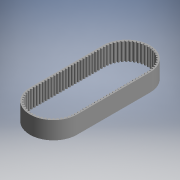
# Autodesk Inventor part: SLZ_63_Riemen#
Saved by Autodesk Inventor 2017.3 (Build 213256000, 256)
## iProperties
Part Number: SLZ_63_Riemen#
Material: Generic
Catalog Web Link: www.cadenas.de
Description: Riemen_SLZ63-Control-Tec
Vendor: ROSEKRIEGER
Document SubType Name: Modeling
Designer: partserver
Manufacturer: ROSEKRIEGER
Mass: 50.6703 g
Surface Area: 430.175 cm^2
Volume: 50.6703 cm^3
Density: 1 g/cm^3
Appearance: PSOLRGB-191-191-191
Category: PARTsolutions
Company: ROSEKRIEGER
Title: SLZ_63_Riemen#
Author: Cadenas PARTsolutions
Comments: Control-Tec
PSOL_IDENT_0: {$CADENAS_DATA\23d-libs\rose_krieger\linearkomponenten\pool_lineartechnik\_hubsaeule_zyliinder\elekt
PSOL_IDENT_1: rozylinder\elekzyl_slz63\parts\slz63_plfl_antrieb_riemen.prj},174 {VTYP=3D},{NB=SLZ_63_Riemen#},{LIN
PSOL_IDENT_2: A=SLZ_63_Riemen#},{NN=Riemen_SLZ63},{DATE=02.12.2020 11:16:24},{GEOMDATE=22.06.2016 13:11:00},{VERSI
PSOL_IDENT_3: ON=},{LINEID=10},{WBVAR=},{WBNUMERIC=}  {NB=SLZ_63_Riemen#},{LINA=SLZ_63_Riemen#},{KT=DUMMY},{IDNR=}
PSOL_IDENT_4: ,{CODE=TQ3},{ARTIKEL=Elektrozylinder },{TYPE=SLZ 63 KG P PL},{BEST=SLZ_63_Riemen},{VARIANTE=PL},{SPI
PSOL_IDENT_5: NDEL=KG 25x10},{SPINDELCODE=3.000},{SCHUTZARTVIS=IP54},{SCHUTZART=1},{HUB1=0,[0:100]},{HINWEINBAUX=H
PSOL_IDENT_6: ub + 288,5 mm},{DUMMYDURCH=10.000},{DUMMYLAENG=20.000},{HILFEHUB=105},{LAENDOPPROFIL=184.500},{RF=1.
PSOL_IDENT_7: 000},{GRUNDKOE=288.500},{A=100},{B=80},{C=100},{D=125},{E=238},{F=40},{G=M16x1.5},{H=104},{K=125},{L=
PSOL_IDENT_8: 105},{M=48},{N=56.5},{O=86},{P=18.5},{PPATH=sbl_lz70p_plfl.prj}
NB: SLZ_63_Riemen#
NN: Riemen_SLZ63
NT: Control-Tec
NBSYN: $BEST.#
LINA: SLZ_63_Riemen#
CATALOG: RK Rose+Krieger
ARTIKEL: Elektrozylinder
TYPE: SLZ 63 KG P PL
BEST: SLZ_63_Riemen
VARIANTE: PL
SPINDEL: KG 25x10
SPINDELCODE: 3
SCHUTZARTVIS: IP54
SCHUTZART: 1
HUB1: 0,[0:100]
HINWEINBAUX: Hub + 288,5 mm
DUMMYDURCH: 10
DUMMYLAENG: 20
HILFEHUB: 105
LAENDOPPROFIL: 184.5
RF: 1
GRUNDKOE: 288.5
A: 100
B: 80
C: 100
D: 125
E: 238
F: 40
G: M16x1.5
H: 104
K: 125
L: 105
M: 48
N: 56.5
O: 86
P: 18.5
SUPPLIER: ROSEKRIEGER
ARTICLENO: SLZ_63_Riemen#
BOMINFO: SLZ_63_Riemen#
CREATOR: CADENAS GmbH
Autodesk Inventor part; units mm, degrees
sketch "Sketch_2" plane through (0, 0, 0) normal (0, 0, 1) x (1, 0, 0)
  arc A0 (-40.2, -125) -> (40.2, -125) centre (0, -125) ccw
  line L0 (40.2, -125) -> (40.2, 0)
  arc A1 (40.2, 0) -> (-40.2, 0) centre (0, 0) ccw
  line L1 (-40.2, 0) -> (-40.2, -125)
  arc A2 (-38.1613, -126.7182) -> (-38.195, -123.2926) centre (-37.625, -125) ccw
  arc A3 (-38.1613, -126.7182) -> (-38.0591, -128.2775) centre (0, -125) ccw
  arc A4 (-37.6106, -131.6846) -> (-38.0591, -128.2775) centre (-37.3031, -129.911) ccw
  arc A5 (-37.6106, -131.6846) -> (-37.3057, -133.2172) centre (0, -125) ccw
  arc A6 (-36.4163, -136.5366) -> (-37.3057, -133.2172) centre (-36.343, -134.7381) ccw
  arc A7 (-36.4163, -136.5366) -> (-35.914, -138.0163) centre (0, -125) ccw
  arc A8 (-34.5989, -141.1912) -> (-35.914, -138.0163) centre (-34.761, -139.3985) ccw
  arc A9 (-34.5989, -141.1912) -> (-33.9078, -142.5926) centre (0, -125) ccw
  arc A10 (-32.1896, -145.5687) -> (-33.9078, -142.5926) centre (-32.5842, -143.8125) ccw
  arc A11 (-32.1896, -145.5687) -> (-31.3214, -146.868) centre (0, -125) ccw
  arc A12 (-29.2294, -149.5943) -> (-31.3214, -146.868) centre (-29.8499, -147.9046) ccw
  arc A13 (-29.2294, -149.5943) -> (-28.1991, -150.7692) centre (0, -125) ccw
  arc A14 (-25.7692, -153.1991) -> (-28.1991, -150.7692) centre (-26.6049, -151.6049) ccw
  arc A15 (-25.7692, -153.1991) -> (-24.5943, -154.2294) centre (0, -125) ccw
  arc A16 (-21.868, -156.3214) -> (-24.5943, -154.2294) centre (-22.9046, -154.8499) ccw
  arc A17 (-21.868, -156.3214) -> (-20.5687, -157.1896) centre (0, -125) ccw
  arc A18 (-17.5926, -158.9078) -> (-20.5687, -157.1896) centre (-18.8125, -157.5842) ccw
  arc A19 (-17.5926, -158.9078) -> (-16.1912, -159.5989) centre (0, -125) ccw
  arc A20 (-13.0163, -160.914) -> (-16.1912, -159.5989) centre (-14.3985, -159.761) ccw
  arc A21 (-13.0163, -160.914) -> (-11.5366, -161.4163) centre (0, -125) ccw
  arc A22 (-8.2172, -162.3057) -> (-11.5366, -161.4163) centre (-9.7381, -161.343) ccw
  arc A23 (-8.2172, -162.3057) -> (-6.6846, -162.6106) centre (0, -125) ccw
  arc A24 (-3.2775, -163.0591) -> (-6.6846, -162.6106) centre (-4.911, -162.3031) ccw
  arc A25 (-3.2775, -163.0591) -> (-1.7182, -163.1613) centre (0, -125) ccw
  arc A26 (1.7182, -163.1613) -> (-1.7182, -163.1613) centre (0, -162.625) ccw
  arc A27 (1.7182, -163.1613) -> (3.2775, -163.0591) centre (0, -125) ccw
  arc A28 (6.6846, -162.6106) -> (3.2775, -163.0591) centre (4.911, -162.3031) ccw
  arc A29 (6.6846, -162.6106) -> (8.2172, -162.3057) centre (0, -125) ccw
  arc A30 (11.5366, -161.4163) -> (8.2172, -162.3057) centre (9.7381, -161.343) ccw
  arc A31 (11.5366, -161.4163) -> (13.0163, -160.914) centre (0, -125) ccw
  arc A32 (16.1912, -159.5989) -> (13.0163, -160.914) centre (14.3985, -159.761) ccw
  arc A33 (16.1912, -159.5989) -> (17.5926, -158.9078) centre (0, -125) ccw
  arc A34 (20.5687, -157.1896) -> (17.5926, -158.9078) centre (18.8125, -157.5842) ccw
  arc A35 (20.5687, -157.1896) -> (21.868, -156.3214) centre (0, -125) ccw
  arc A36 (24.5943, -154.2294) -> (21.868, -156.3214) centre (22.9046, -154.8499) ccw
  arc A37 (24.5943, -154.2294) -> (25.7692, -153.1991) centre (0, -125) ccw
  arc A38 (28.1991, -150.7692) -> (25.7692, -153.1991) centre (26.6049, -151.6049) ccw
  arc A39 (28.1991, -150.7692) -> (29.2294, -149.5943) centre (0, -125) ccw
  arc A40 (31.3214, -146.868) -> (29.2294, -149.5943) centre (29.8499, -147.9046) ccw
  arc A41 (31.3214, -146.868) -> (32.1896, -145.5687) centre (0, -125) ccw
  arc A42 (33.9078, -142.5926) -> (32.1896, -145.5687) centre (32.5842, -143.8125) ccw
  arc A43 (33.9078, -142.5926) -> (34.5989, -141.1912) centre (0, -125) ccw
  arc A44 (35.914, -138.0163) -> (34.5989, -141.1912) centre (34.761, -139.3985) ccw
  arc A45 (35.914, -138.0163) -> (36.4163, -136.5366) centre (0, -125) ccw
  arc A46 (37.3057, -133.2172) -> (36.4163, -136.5366) centre (36.343, -134.7381) ccw
  arc A47 (37.3057, -133.2172) -> (37.6106, -131.6846) centre (0, -125) ccw
  arc A48 (38.0591, -128.2775) -> (37.6106, -131.6846) centre (37.3031, -129.911) ccw
  arc A49 (38.0591, -128.2775) -> (38.1613, -126.7182) centre (0, -125) ccw
  arc A50 (38.195, -123.2926) -> (38.1613, -126.7182) centre (37.625, -125) ccw
  line L2 (38.195, -123.2926) -> (38.195, -121.7074)
  arc A51 (38.195, -118.2926) -> (38.195, -121.7074) centre (37.625, -120) ccw
  line L3 (38.195, -118.2926) -> (38.195, -116.7074)
  arc A52 (38.195, -113.2926) -> (38.195, -116.7074) centre (37.625, -115) ccw
  line L4 (38.195, -113.2926) -> (38.195, -111.7074)
  arc A53 (38.195, -108.2926) -> (38.195, -111.7074) centre (37.625, -110) ccw
  line L5 (38.195, -108.2926) -> (38.195, -106.7074)
  arc A54 (38.195, -103.2926) -> (38.195, -106.7074) centre (37.625, -105) ccw
  line L6 (38.195, -103.2926) -> (38.195, -101.7074)
  arc A55 (38.195, -98.2926) -> (38.195, -101.7074) centre (37.625, -100) ccw
  line L7 (38.195, -98.2926) -> (38.195, -96.7074)
  arc A56 (38.195, -93.2926) -> (38.195, -96.7074) centre (37.625, -95) ccw
  line L8 (38.195, -93.2926) -> (38.195, -91.7074)
  arc A57 (38.195, -88.2926) -> (38.195, -91.7074) centre (37.625, -90) ccw
  line L9 (38.195, -88.2926) -> (38.195, -86.7074)
  arc A58 (38.195, -83.2926) -> (38.195, -86.7074) centre (37.625, -85) ccw
  line L10 (38.195, -83.2926) -> (38.195, -81.7074)
  arc A59 (38.195, -78.2926) -> (38.195, -81.7074) centre (37.625, -80) ccw
  line L11 (38.195, -78.2926) -> (38.195, -76.7074)
  arc A60 (38.195, -73.2926) -> (38.195, -76.7074) centre (37.625, -75) ccw
  line L12 (38.195, -73.2926) -> (38.195, -71.7074)
  arc A61 (38.195, -68.2926) -> (38.195, -71.7074) centre (37.625, -70) ccw
  line L13 (38.195, -68.2926) -> (38.195, -66.7074)
  arc A62 (38.195, -63.2926) -> (38.195, -66.7074) centre (37.625, -65) ccw
  line L14 (38.195, -63.2926) -> (38.195, -61.7074)
  arc A63 (38.195, -58.2926) -> (38.195, -61.7074) centre (37.625, -60) ccw
  line L15 (38.195, -58.2926) -> (38.195, -56.7074)
  arc A64 (38.195, -53.2926) -> (38.195, -56.7074) centre (37.625, -55) ccw
  line L16 (38.195, -53.2926) -> (38.195, -51.7074)
  arc A65 (38.195, -48.2926) -> (38.195, -51.7074) centre (37.625, -50) ccw
  line L17 (38.195, -48.2926) -> (38.195, -46.7074)
  arc A66 (38.195, -43.2926) -> (38.195, -46.7074) centre (37.625, -45) ccw
  line L18 (38.195, -43.2926) -> (38.195, -41.7074)
  arc A67 (38.195, -38.2926) -> (38.195, -41.7074) centre (37.625, -40) ccw
  line L19 (38.195, -38.2926) -> (38.195, -36.7074)
  arc A68 (38.195, -33.2926) -> (38.195, -36.7074) centre (37.625, -35) ccw
  line L20 (38.195, -33.2926) -> (38.195, -31.7074)
  arc A69 (38.195, -28.2926) -> (38.195, -31.7074) centre (37.625, -30) ccw
  line L21 (38.195, -28.2926) -> (38.195, -26.7074)
  arc A70 (38.195, -23.2926) -> (38.195, -26.7074) centre (37.625, -25) ccw
  line L22 (38.195, -23.2926) -> (38.195, -21.7074)
  arc A71 (38.195, -18.2926) -> (38.195, -21.7074) centre (37.625, -20) ccw
  line L23 (38.195, -18.2926) -> (38.195, -16.7074)
  arc A72 (38.195, -13.2926) -> (38.195, -16.7074) centre (37.625, -15) ccw
  line L24 (38.195, -13.2926) -> (38.195, -11.7074)
  arc A73 (38.195, -8.2926) -> (38.195, -11.7074) centre (37.625, -10) ccw
  line L25 (38.195, -8.2926) -> (38.195, -6.7074)
  arc A74 (38.195, -3.2926) -> (38.195, -6.7074) centre (37.625, -5) ccw
  line L26 (38.195, -3.2926) -> (38.195, -1.7074)
  arc A75 (38.1613, 1.7182) -> (38.195, -1.7074) centre (37.625, 0) ccw
  arc A76 (38.1613, 1.7182) -> (38.0591, 3.2775) centre (0, 0) ccw
  arc A77 (37.6106, 6.6846) -> (38.0591, 3.2775) centre (37.3031, 4.911) ccw
  arc A78 (37.6106, 6.6846) -> (37.3057, 8.2172) centre (0, 0) ccw
  arc A79 (36.4163, 11.5366) -> (37.3057, 8.2172) centre (36.343, 9.7381) ccw
  arc A80 (36.4163, 11.5366) -> (35.914, 13.0163) centre (0, 0) ccw
  arc A81 (34.5989, 16.1912) -> (35.914, 13.0163) centre (34.761, 14.3985) ccw
  arc A82 (34.5989, 16.1912) -> (33.9078, 17.5926) centre (0, 0) ccw
  arc A83 (32.1896, 20.5687) -> (33.9078, 17.5926) centre (32.5842, 18.8125) ccw
  arc A84 (32.1896, 20.5687) -> (31.3214, 21.868) centre (0, 0) ccw
  arc A85 (29.2294, 24.5943) -> (31.3214, 21.868) centre (29.8499, 22.9046) ccw
  arc A86 (29.2294, 24.5943) -> (28.1991, 25.7692) centre (0, 0) ccw
  arc A87 (25.7692, 28.1991) -> (28.1991, 25.7692) centre (26.6049, 26.6049) ccw
  arc A88 (25.7692, 28.1991) -> (24.5943, 29.2294) centre (0, 0) ccw
  arc A89 (21.868, 31.3214) -> (24.5943, 29.2294) centre (22.9046, 29.8499) ccw
  arc A90 (21.868, 31.3214) -> (20.5687, 32.1896) centre (0, 0) ccw
  arc A91 (17.5926, 33.9078) -> (20.5687, 32.1896) centre (18.8125, 32.5842) ccw
  arc A92 (17.5926, 33.9078) -> (16.1912, 34.5989) centre (0, 0) ccw
  arc A93 (13.0163, 35.914) -> (16.1912, 34.5989) centre (14.3985, 34.761) ccw
  arc A94 (13.0163, 35.914) -> (11.5366, 36.4163) centre (0, 0) ccw
  arc A95 (8.2172, 37.3057) -> (11.5366, 36.4163) centre (9.7381, 36.343) ccw
  arc A96 (8.2172, 37.3057) -> (6.6846, 37.6106) centre (0, 0) ccw
  arc A97 (3.2775, 38.0591) -> (6.6846, 37.6106) centre (4.911, 37.3031) ccw
  arc A98 (3.2775, 38.0591) -> (1.7182, 38.1613) centre (0, 0) ccw
  arc A99 (-1.7182, 38.1613) -> (1.7182, 38.1613) centre (0, 37.625) ccw
  arc A100 (-1.7182, 38.1613) -> (-3.2775, 38.0591) centre (0, 0) ccw
  arc A101 (-6.6846, 37.6106) -> (-3.2775, 38.0591) centre (-4.911, 37.3031) ccw
  arc A102 (-6.6846, 37.6106) -> (-8.2172, 37.3057) centre (0, 0) ccw
  arc A103 (-11.5366, 36.4163) -> (-8.2172, 37.3057) centre (-9.7381, 36.343) ccw
  arc A104 (-11.5366, 36.4163) -> (-13.0163, 35.914) centre (0, 0) ccw
  arc A105 (-16.1912, 34.5989) -> (-13.0163, 35.914) centre (-14.3985, 34.761) ccw
  arc A106 (-16.1912, 34.5989) -> (-17.5926, 33.9078) centre (0, 0) ccw
  arc A107 (-20.5687, 32.1896) -> (-17.5926, 33.9078) centre (-18.8125, 32.5842) ccw
  arc A108 (-20.5687, 32.1896) -> (-21.868, 31.3214) centre (0, 0) ccw
  arc A109 (-24.5943, 29.2294) -> (-21.868, 31.3214) centre (-22.9046, 29.8499) ccw
  arc A110 (-24.5943, 29.2294) -> (-25.7692, 28.1991) centre (0, 0) ccw
  arc A111 (-28.1991, 25.7692) -> (-25.7692, 28.1991) centre (-26.6049, 26.6049) ccw
  arc A112 (-28.1991, 25.7692) -> (-29.2294, 24.5943) centre (0, 0) ccw
  arc A113 (-31.3214, 21.868) -> (-29.2294, 24.5943) centre (-29.8499, 22.9046) ccw
  arc A114 (-31.3214, 21.868) -> (-32.1896, 20.5687) centre (0, 0) ccw
  arc A115 (-33.9078, 17.5926) -> (-32.1896, 20.5687) centre (-32.5842, 18.8125) ccw
  arc A116 (-33.9078, 17.5926) -> (-34.5989, 16.1912) centre (0, 0) ccw
  arc A117 (-35.914, 13.0163) -> (-34.5989, 16.1912) centre (-34.761, 14.3985) ccw
  arc A118 (-35.914, 13.0163) -> (-36.4163, 11.5366) centre (0, 0) ccw
  arc A119 (-37.3057, 8.2172) -> (-36.4163, 11.5366) centre (-36.343, 9.7381) ccw
  arc A120 (-37.3057, 8.2172) -> (-37.6106, 6.6846) centre (0, 0) ccw
  arc A121 (-38.0591, 3.2775) -> (-37.6106, 6.6846) centre (-37.3031, 4.911) ccw
  arc A122 (-38.0591, 3.2775) -> (-38.1613, 1.7182) centre (0, 0) ccw
  arc A123 (-38.195, -1.7074) -> (-38.1613, 1.7182) centre (-37.625, 0) ccw
  line L27 (-38.195, -1.7074) -> (-38.195, -3.2926)
  arc A124 (-38.195, -6.7074) -> (-38.195, -3.2926) centre (-37.625, -5) ccw
  line L28 (-38.195, -6.7074) -> (-38.195, -8.2926)
  arc A125 (-38.195, -11.7074) -> (-38.195, -8.2926) centre (-37.625, -10) ccw
  line L29 (-38.195, -11.7074) -> (-38.195, -13.2926)
  arc A126 (-38.195, -16.7074) -> (-38.195, -13.2926) centre (-37.625, -15) ccw
  line L30 (-38.195, -16.7074) -> (-38.195, -18.2926)
  arc A127 (-38.195, -21.7074) -> (-38.195, -18.2926) centre (-37.625, -20) ccw
  line L31 (-38.195, -21.7074) -> (-38.195, -23.2926)
  arc A128 (-38.195, -26.7074) -> (-38.195, -23.2926) centre (-37.625, -25) ccw
  line L32 (-38.195, -26.7074) -> (-38.195, -28.2926)
  arc A129 (-38.195, -31.7074) -> (-38.195, -28.2926) centre (-37.625, -30) ccw
  line L33 (-38.195, -31.7074) -> (-38.195, -33.2926)
  arc A130 (-38.195, -36.7074) -> (-38.195, -33.2926) centre (-37.625, -35) ccw
  line L34 (-38.195, -36.7074) -> (-38.195, -38.2926)
  arc A131 (-38.195, -41.7074) -> (-38.195, -38.2926) centre (-37.625, -40) ccw
  line L35 (-38.195, -41.7074) -> (-38.195, -43.2926)
  arc A132 (-38.195, -46.7074) -> (-38.195, -43.2926) centre (-37.625, -45) ccw
  line L36 (-38.195, -46.7074) -> (-38.195, -48.2926)
  arc A133 (-38.195, -51.7074) -> (-38.195, -48.2926) centre (-37.625, -50) ccw
  line L37 (-38.195, -51.7074) -> (-38.195, -53.2926)
  arc A134 (-38.195, -56.7074) -> (-38.195, -53.2926) centre (-37.625, -55) ccw
  line L38 (-38.195, -56.7074) -> (-38.195, -58.2926)
  arc A135 (-38.195, -61.7074) -> (-38.195, -58.2926) centre (-37.625, -60) ccw
  line L39 (-38.195, -61.7074) -> (-38.195, -63.2926)
  arc A136 (-38.195, -66.7074) -> (-38.195, -63.2926) centre (-37.625, -65) ccw
  line L40 (-38.195, -66.7074) -> (-38.195, -68.2926)
  arc A137 (-38.195, -71.7074) -> (-38.195, -68.2926) centre (-37.625, -70) ccw
  line L41 (-38.195, -71.7074) -> (-38.195, -73.2926)
  arc A138 (-38.195, -76.7074) -> (-38.195, -73.2926) centre (-37.625, -75) ccw
  line L42 (-38.195, -76.7074) -> (-38.195, -78.2926)
  arc A139 (-38.195, -81.7074) -> (-38.195, -78.2926) centre (-37.625, -80) ccw
  line L43 (-38.195, -81.7074) -> (-38.195, -83.2926)
  arc A140 (-38.195, -86.7074) -> (-38.195, -83.2926) centre (-37.625, -85) ccw
  line L44 (-38.195, -86.7074) -> (-38.195, -88.2926)
  arc A141 (-38.195, -91.7074) -> (-38.195, -88.2926) centre (-37.625, -90) ccw
  line L45 (-38.195, -91.7074) -> (-38.195, -93.2926)
  arc A142 (-38.195, -96.7074) -> (-38.195, -93.2926) centre (-37.625, -95) ccw
  line L46 (-38.195, -96.7074) -> (-38.195, -98.2926)
  arc A143 (-38.195, -101.7074) -> (-38.195, -98.2926) centre (-37.625, -100) ccw
  line L47 (-38.195, -101.7074) -> (-38.195, -103.2926)
  arc A144 (-38.195, -106.7074) -> (-38.195, -103.2926) centre (-37.625, -105) ccw
  line L48 (-38.195, -106.7074) -> (-38.195, -108.2926)
  arc A145 (-38.195, -111.7074) -> (-38.195, -108.2926) centre (-37.625, -110) ccw
  line L49 (-38.195, -111.7074) -> (-38.195, -113.2926)
  arc A146 (-38.195, -116.7074) -> (-38.195, -113.2926) centre (-37.625, -115) ccw
  line L50 (-38.195, -116.7074) -> (-38.195, -118.2926)
  arc A147 (-38.195, -121.7074) -> (-38.195, -118.2926) centre (-37.625, -120) ccw
  line L51 (-38.195, -121.7074) -> (-38.195, -123.2926)
  constraints: 296 point on circle, 148 centre point, 104 end point
extrude "Extrusion1" add sketch "Sketch_2" along normal blind 30
ref_plane "RIEMEN_XY" through (0, 0, 15) normal (0, 0, -1) x (1, 0, 0)
ref_plane "RIEMEN_YZ" through (0, 0, 15) normal (1, 0, 0) x (0, -1, 0)
ref_plane "RIEMEN_ZX" through (0, 0, 15) normal (0, -1, 0) x (0, 0, -1)
body "Solid1"
